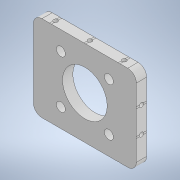
# Autodesk Inventor part: エアシリンダマウント
Saved by Autodesk Inventor 2021 (Build 250183000, 183)
## iProperties
Created: 2022-02-01
Part Number: エアシリンダマウント
Material: 一般
Document SubType Name: Modeling
Designer: hirohumi
Density: 1 g/cm^3
Appearance: 既定
Author: hirohumi
Autodesk Inventor part; units mm, degrees
ref_plane "YZ Plane" through (0, 0, 0) normal (1, 0, 0) x (0, 1, 0)
ref_plane "XZ Plane" through (0, 0, 0) normal (0, 1, 0) x (-1, 0, 0)
ref_plane "XY Plane" through (0, 0, 0) normal (0, 0, 1) x (1, 0, 0)
sketch "スケッチ1" plane through (0, 0, 0) normal (0, 0, 1) x (1, 0, 0)
  circle A0 centre (0, 0) radius 13
  circle A1 centre (-14, 14) radius 2.6
  circle A2 centre (14, 14) radius 2.6
  circle A3 centre (14, -14) radius 2.6
  circle A4 centre (-14, -14) radius 2.6
  line L0 (25, 25) -> (20.5385, 25)
  line L1 (-30, 20) -> (-30, 8.0385)
  line L2 (-25, -25) -> (-20.5385, -25)
  line L3 (30, -20) -> (30, -8.0385)
  line L4 (30, 25) -> (-30, -25) construction
  line L5 (-30, 25) -> (30, -25) construction
  arc A5 (-19.4615, 25) -> (-20.5385, 25) centre (-20, 26.4) ccw construction
  arc A6 (0.5385, 25) -> (-0.5385, 25) centre (0, 26.4) ccw construction
  arc A7 (20.5385, 25) -> (19.4615, 25) centre (20, 26.4) ccw construction
  arc A8 (-20.5385, 25) -> (-19.4615, 25) centre (-20, 26.4) ccw
  line L6 (-19.4615, 25) -> (-20.5385, 25) construction
  line L7 (-20.5385, 25) -> (-25, 25)
  arc A9 (-0.5385, 25) -> (0.5385, 25) centre (0, 26.4) ccw
  line L8 (0.5385, 25) -> (-0.5385, 25) construction
  line L9 (-0.5385, 25) -> (-19.4615, 25)
  arc A10 (19.4615, 25) -> (20.5385, 25) centre (20, 26.4) ccw
  line L10 (20.5385, 25) -> (19.4615, 25) construction
  line L11 (19.4615, 25) -> (0.5385, 25)
  arc A11 (-0.5385, -25) -> (0.5385, -25) centre (0, -26.4) ccw construction
  arc A12 (-20.5385, -25) -> (-19.4615, -25) centre (-20, -26.4) ccw construction
  arc A13 (19.4615, -25) -> (20.5385, -25) centre (20, -26.4) ccw construction
  arc A14 (-19.4615, -25) -> (-20.5385, -25) centre (-20, -26.4) ccw
  line L12 (-19.4615, -25) -> (-0.5385, -25)
  line L13 (-20.5385, -25) -> (-19.4615, -25) construction
  arc A15 (0.5385, -25) -> (-0.5385, -25) centre (0, -26.4) ccw
  line L14 (0.5385, -25) -> (19.4615, -25)
  line L15 (-0.5385, -25) -> (0.5385, -25) construction
  arc A16 (20.5385, -25) -> (19.4615, -25) centre (20, -26.4) ccw
  line L16 (20.5385, -25) -> (25, -25)
  line L17 (19.4615, -25) -> (20.5385, -25) construction
  arc A17 (-30, 8.0385) -> (-30, 6.9615) centre (-31.4, 7.5) ccw construction
  arc A18 (-30, -6.9615) -> (-30, -8.0385) centre (-31.4, -7.5) ccw construction
  arc A19 (30, 6.9615) -> (30, 8.0385) centre (31.4, 7.5) ccw construction
  arc A20 (30, -8.0385) -> (30, -6.9615) centre (31.4, -7.5) ccw construction
  arc A21 (-30, 6.9615) -> (-30, 8.0385) centre (-31.4, 7.5) ccw
  line L18 (-30, 6.9615) -> (-30, -6.9615)
  line L19 (-30, 8.0385) -> (-30, 6.9615) construction
  arc A22 (-30, -8.0385) -> (-30, -6.9615) centre (-31.4, -7.5) ccw
  line L20 (-30, -8.0385) -> (-30, -20)
  line L21 (-30, -6.9615) -> (-30, -8.0385) construction
  arc A23 (30, 8.0385) -> (30, 6.9615) centre (31.4, 7.5) ccw
  line L22 (30, 6.9615) -> (30, 8.0385) construction
  line L23 (30, 8.0385) -> (30, 20)
  arc A24 (30, -6.9615) -> (30, -8.0385) centre (31.4, -7.5) ccw
  line L24 (30, -6.9615) -> (30, 6.9615)
  line L25 (30, -8.0385) -> (30, -6.9615) construction
  arc A25 (-25, 25) -> (-30, 20) centre (-25, 20) ccw
  arc A26 (30, 20) -> (25, 25) centre (25, 20) ccw
  arc A27 (25, -25) -> (30, -20) centre (25, -20) ccw
  arc A28 (-30, -20) -> (-25, -25) centre (-25, -20) ccw
  point P0 (0, 0)
  point P1 (0, 0)
  dimension "d0" = 26
  dimension "d1" = 28
  dimension "d2" = 14
  dimension "d3" = 5.2
  dimension "d4" = 5.2
  dimension "d5" = 28
  dimension "d6" = 14
  dimension "d7" = 5.2
  dimension "d8" = 5.2
  dimension "d9" = 60
  dimension "d10" = 50
  dimension "d11" = 3
  dimension "d12" = 3
  dimension "d13" = 20
  dimension "d14" = 3
  dimension "d15" = 20
  dimension "d16" = 1.4
  dimension "d17" = 3
  dimension "d18" = 3
  dimension "d19" = 3
  dimension "d20" = 20
  dimension "d21" = 20
  dimension "d22" = 1.4
  dimension "d23" = 3
  dimension "d24" = 3
  dimension "d25" = 3
  dimension "d26" = 3
  dimension "d27" = 15
  dimension "d28" = 15
  dimension "d29" = 7.5
  dimension "d30" = 7.5
  dimension "d31" = 1.4
  dimension "d32" = 1.4
  dimension "d33" = 5
  constraints: 74 parallel, 52 end point, 48 point on circle, 35 perpendicular, 29 centre point, 12 point on line, 8 tangent, 7 horizontal, 6 horizontal alignment, 6 vertical alignment, 4 midpoint, 3 equal radius, 1 coincident
  measures "d0" diameter of A0
  measures "d1" distance of A2.centre A1.centre
  measures "d2" horizontal distance of point (0, 0) A1.centre
  measures "d3" diameter of A1
  measures "d4" diameter of A2
  measures "d5" distance of A4.centre A1.centre
  measures "d6" horizontal distance of point (0, 0) A1.centre
  measures "d7" diameter of A4
  measures "d8" diameter of A3
  measures "d9" distance of L4.start L5.start
  measures "d10" distance of L5.start L4.end
  measures "d11" diameter of A5
  measures "d12" diameter of A6
  measures "d13" distance of A6.centre A5.centre
  measures "d14" diameter of A7
  measures "d15" distance of A7.centre A6.centre
  measures "d16" distance from line of L0 A6.centre
  measures "d17" diameter of A11
  measures "d18" diameter of A12
  measures "d19" diameter of A13
  measures "d20" distance of A11.centre A12.centre
  measures "d21" distance of A13.centre A11.centre
  measures "d22" distance from line of L2 A11.centre
  measures "d23" diameter of A17
  measures "d24" diameter of A18
  measures "d25" diameter of A19
  measures "d26" diameter of A20
  measures "d27" distance of A18.centre A17.centre
  measures "d28" distance of A20.centre A19.centre
  measures "d29" vertical distance of A0.centre A17.centre
  measures "d30" vertical distance of point (0, 0) A19.centre
  measures "d31" distance from line of L1 A17.centre
  measures "d32" distance from line of L3 A19.centre
  measures "d33" radius of A25
extrude "押し出し1" add sketch "スケッチ1" along normal blind 6
sketch "スケッチ2" plane through (-19.4615, 25, 0) normal (0, 1, 0) x (1, 0, 0)
  circle A0 centre (-0.5385, -3) radius 1.25
  circle A1 centre (19.4615, -3) radius 1.25
  circle A2 centre (39.4615, -3) radius 1.25
  point P0 (19.4615, 0)
  dimension "d36" = 2.5
  dimension "d37" = 2.5
  dimension "d38" = 2.5
  dimension "d39" = 3
  dimension "d40" = 20
  dimension "d41" = 20
  constraints: 3 centre point, 2 horizontal alignment, 1 vertical alignment
  measures "d36" diameter of A0
  measures "d37" diameter of A1
  measures "d38" diameter of A2
  measures "d39" distance of point (19.461, 0) A1.centre
  measures "d40" distance of A1.centre A0.centre
  measures "d41" distance of A2.centre A1.centre
sketch "スケッチ3" plane through (30, -6.9615, 0) normal (1, 0, 0) x (0, 0, -1)
  circle A0 centre (-3, 14.4615) radius 1.25
  circle A1 centre (-3, -0.5385) radius 1.25
  point P0 (0, 6.9615)
  dimension "d42" = 2.5
  dimension "d43" = 2.5
  dimension "d44" = 3
  dimension "d45" = 7.5
  dimension "d46" = 7.5
  constraints: 2 centre point, 1 vertical alignment
  measures "d42" diameter of A0
  measures "d43" diameter of A1
  measures "d44" horizontal distance of point (0, 6.961) A0.centre
  measures "d45" vertical distance of A0.centre point (0, 6.961)
  measures "d46" vertical distance of point (0, 6.961) A1.centre
extrude "押し出し2" cut sketch "スケッチ3" against normal blind 10
extrude "押し出し3" cut sketch "スケッチ2" against normal blind 10
sketch "スケッチ4" plane through (0.5385, -25, 0) normal (0, -1, 0) x (1, 0, 0)
  circle A0 centre (-0.5385, 3) radius 1.25
  circle A1 centre (-20.5385, 3) radius 1.25
  circle A2 centre (19.4615, 3) radius 1.25
  point P0 (-0.5385, 0)
  dimension "d51" = 2.5
  dimension "d52" = 2.5
  dimension "d53" = 2.5
  dimension "d54" = 20
  dimension "d55" = 20
  dimension "d56" = 3
  constraints: 3 centre point, 2 horizontal alignment, 1 vertical alignment
  measures "d51" diameter of A0
  measures "d52" diameter of A1
  measures "d53" diameter of A2
  measures "d54" distance of A0.centre A1.centre
  measures "d55" distance of A2.centre A0.centre
  measures "d56" distance of point (-0.539, 0) A0.centre
extrude "押し出し4" cut sketch "スケッチ4" against normal blind 10
sketch "スケッチ5" plane through (-30, -6.9615, 0) normal (-1, 0, 0) x (0, 0, 1)
  circle A0 centre (3, 14.4615) radius 1.25 projected
  circle A1 centre (3, -0.5385) radius 1.25 projected
  point P0 (0, 6.9615)
extrude "押し出し5" cut sketch "スケッチ5" against normal blind 10
equation "\"d2\" = 0.5 * d1"
equation "\"d6\" = 0.5 * d5"
equation "\"d29\" = 0.5 * d27"
equation "\"d30\" = 0.5 * d28"
